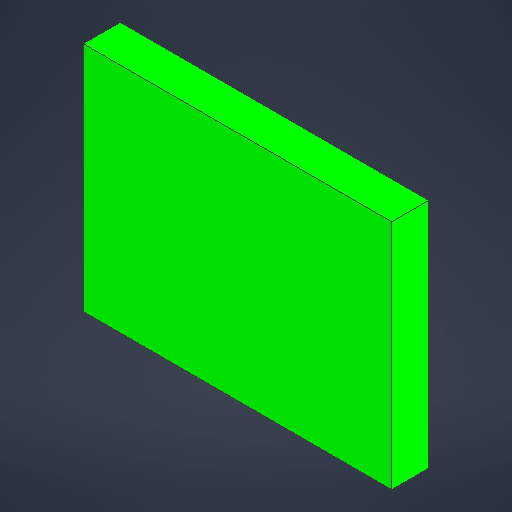
# Autodesk Inventor part: insulation2
Saved by Autodesk Inventor 2025.2 (Build 292293000, 293)
## iProperties
Created: 2025-03-05
Part Number: insulation2
Material: Generic
Document SubType Name: Modeling
Designer: cbast
Density: 1 g/cm^3
Appearance: Default
Author: cbast
Autodesk Inventor part; units mm, degrees
ref_plane "YZ Plane" through (0, 0, 0) normal (1, 0, 0) x (0, 1, 0)
ref_plane "XZ Plane" through (0, 0, 0) normal (0, 1, 0) x (-1, 0, 0)
ref_plane "XY Plane" through (0, 0, 0) normal (0, 0, 1) x (1, 0, 0)
sketch "Sketch1" plane through (0, 0, 0) normal (0, 0, 1) x (1, 0, 0)
  line L0 (77.2, 10.9497) -> (83.8464, 10.9497) projected
  line L1 (83.8464, 10.9497) -> (83.8464, 62.15) projected
  line L2 (83.8464, 62.15) -> (-82.8464, 62.15) projected
  line L3 (-82.8464, 62.15) -> (-82.8464, 10.9497) projected
  line L4 (-82.8464, 10.9497) -> (-76.2, 10.9497) projected
  line L5 (-76.2, 10.9497) -> (-76.2, 57.15) projected
  line L6 (-76.2, 57.15) -> (77.2, 57.15) projected
  line L7 (77.2, 57.15) -> (77.2, 10.9497) projected
  line L8 (83.8464, -12.0497) -> (77.2, -12.0497) projected
  line L9 (77.2, -12.0497) -> (77.2, -58.25) projected
  line L10 (77.2, -58.25) -> (-76.2, -58.25) projected
  line L11 (-76.2, -58.25) -> (-76.2, -12.0497) projected
  line L12 (-76.2, -12.0497) -> (-82.8464, -12.0497) projected
  line L13 (-82.8464, -12.0497) -> (-82.8464, -63.25) projected
  line L14 (-82.8464, -63.25) -> (83.8464, -63.25) projected
  line L15 (83.8464, -63.25) -> (83.8464, -12.0497) projected
  circle A0 centre (20.5, 16.7705) radius 9.5 projected
  circle A1 centre (0.5, 16.7705) radius 9.5 projected
  line L16 (77.2, 10.9497) -> (77.2, 57.15) projected
  line L17 (77.2, 57.15) -> (-76.2, 57.15) projected
  line L18 (-76.2, 57.15) -> (-76.2, 10.9497) projected
  line L19 (-76.2, 10.9497) -> (-82.8464, 10.9497) projected
  line L20 (-82.8464, -12.0497) -> (-82.8464, 10.9497) projected
  line L21 (-76.2, -12.0497) -> (-82.8464, -12.0497) projected
  line L22 (-76.2, -12.0497) -> (-76.2, -58.25) projected
  line L23 (-76.2, -58.25) -> (77.2, -58.25) projected
  line L24 (77.2, -58.25) -> (77.2, -12.0497) projected
  line L25 (83.8464, -12.0497) -> (77.2, -12.0497) projected
  line L26 (83.8464, 10.9497) -> (83.8464, -12.0497) projected
  line L27 (83.8464, 10.9497) -> (77.2, 10.9497) projected
  circle A2 centre (-19.5, -17.8705) radius 9.5 projected
  circle A3 centre (-68.972, -26.5) radius 3.615 projected
  circle A4 centre (69.972, -26.5) radius 3.615 projected
  circle A5 centre (30.5, -0.55) radius 9.5 projected
  circle A6 centre (-29.5, -0.55) radius 9.5 projected
  circle A7 centre (10.5, -0.55) radius 9.5 projected
  circle A8 centre (-9.5, -0.55) radius 9.5 projected
  circle A9 centre (0.5, -17.8705) radius 9.5 projected
  circle A10 centre (20.5, -17.8705) radius 9.5 projected
  circle A11 centre (-68.972, 25.4) radius 3.615 projected
  circle A12 centre (69.972, 25.4) radius 3.615 projected
  circle A13 centre (-19.5, 16.7705) radius 9.5 projected
  line L28 (-54, -57.15) -> (54, -57.15) projected
  line L29 (54, -57.15) -> (54, 57.15) projected
  line L30 (54, 57.15) -> (-54, 57.15) projected
  line L31 (-54, 57.15) -> (-54, -57.15) projected
  line L32 (-54, -57.15) -> (54, -57.15) projected
  line L33 (54, -57.15) -> (54, 57.15) projected
  line L34 (54, 57.15) -> (-54, 57.15) projected
  line L35 (-54, 57.15) -> (-54, -57.15) projected
  line L36 (1, -0.55) -> (0, -0.55) construction
  line L37 (-82.8464, 62.15) -> (83.8464, 62.15) construction
  line L38 (83.8464, 62.15) -> (83.8464, -63.25) construction
  line L39 (83.8464, -63.25) -> (-82.8464, -63.25) construction
  line L40 (-82.8464, -63.25) -> (-82.8464, 62.15) construction
  line L41 (-82.8464, 62.15) -> (83.8464, -63.25) construction
  line L42 (83.8464, 62.15) -> (-82.8464, -63.25) construction
  line L43 (-82.8464, 62.15) -> (83.8464, 62.15)
  line L44 (83.8464, 62.15) -> (83.8464, -63.25)
  line L45 (83.8464, -63.25) -> (-82.8464, -63.25)
  line L46 (-82.8464, -63.25) -> (-82.8464, 62.15)
  line L47 (-82.8464, 62.15) -> (83.8464, -63.25) construction
  line L48 (83.8464, 62.15) -> (-82.8464, -63.25) construction
  point P0 (0, 0)
  point P1 (0.5, -0.55)
  constraints: 26 end point, 5 midpoint, 4 parallel, 3 horizontal, 2 horizontal alignment, 2 perpendicular, 2 other
extrude "Extrusion1" add sketch "Sketch1" along normal blind 20 contours L7 L6 L5 L4 L3 L2 L1 L0 | L0 L26 L8 L9 L10 L11 L12 L20 L4 L5 L6 L31 L28 L29 L7 | L15 L14 L13 L12 L11 L10 L9 L8 | L29 L28 L31 L6 | A0 | A1 | A2 | A3 | A4 | A5 | A6 | A7 | A8 | A9 | A10 | A11 | A12 | A13
body "Solid1"
